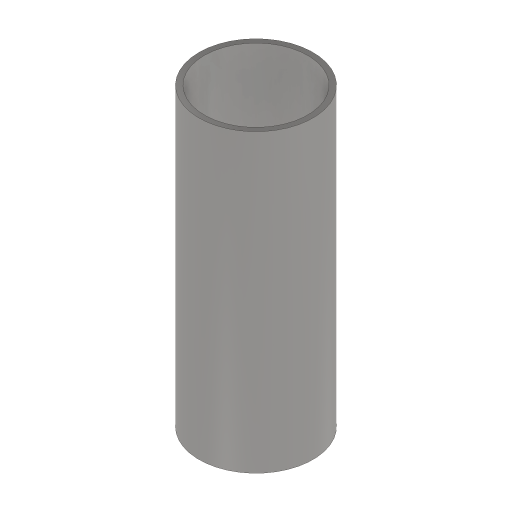
# Autodesk Inventor part: CF70_nipple_Membrane
Saved by Autodesk Inventor 2024.2 (Build 282272000, 272)
## iProperties
Created: 2022-11-16
Part Number: CF70_nipple_Membrane
Material: Stainless Steel, 440C
Document SubType Name: Modeling
Designer: kuzmin
Density: 7.75 g/cm^3
Appearance: Semi-Polished
Mass: 56.0123 g
Surface Area: 146.684 cm^2
Volume: 7.22739 cm^3
Author: kuzmin
Autodesk Inventor part; units mm, degrees
ref_plane "YZ Plane" through (0, 0, 0) normal (1, 0, 0) x (0, 1, 0)
ref_plane "XZ Plane" through (0, 0, 0) normal (0, 1, 0) x (-1, 0, 0)
ref_plane "XY Plane" through (0, 0, 0) normal (0, 0, 1) x (1, 0, 0)
sketch "Sketch1" plane through (0, 0, 0) normal (0, 1, 0) x (-1, 0, 0)
  circle A0 centre (0, 0) radius 19.5
  circle A1 centre (0, 0) radius 21.5
  dimension "d1" = 2
  dimension "d4" = 39
  constraints: 2 centre point, 2 coincident
  measures "d1" radial gap between concentric circles of A0 A1
  measures "d4" diameter of A0
extrude "Extrusion1" add sketch "Sketch1" along normal blind -111.6632
body "Solid1"
